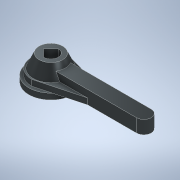
# Autodesk Inventor part: 4-手柄
Saved by Autodesk Inventor 2022 (Build 260153000, 153)
## iProperties
Created: 2023-01-24
Part Number: 4-手柄
Material: 灰口铁
Document SubType Name: Modeling
Designer: Lzy18
Density: 7.15 g/cm^3
Appearance: 灰口铁
Author: Lzy18
Autodesk Inventor part; units mm, degrees
ref_plane "YZ Plane" through (0, 0, 0) normal (1, 0, 0) x (0, 1, 0)
ref_plane "XZ Plane" through (0, 0, 0) normal (0, 1, 0) x (-1, 0, 0)
ref_plane "XY Plane" through (0, 0, 0) normal (0, 0, 1) x (1, 0, 0)
sketch "草图1" plane through (0, 0, 0) normal (0, 1, 0) x (-1, 0, 0)
  arc A0 (0, -13) -> (0, 13) centre (0, 0) ccw
  line L0 (0, 0) -> (-30, 0)
  line L1 (0, -13) -> (-30, -5)
  line L2 (-30, 5) -> (0, 13)
  line L3 (-30, 5) -> (-63, 5)
  line L4 (-63, -5) -> (-30, -5)
  arc A1 (-63, 5) -> (-63, -5) centre (-63, 0) ccw
  dimension "d0" = 26
  dimension "d10" = 10
  constraints: 10 end point, 4 point on circle, 2 centre point, 2 horizontal, 1 coincident, 1 parallel
  measures "d0" diameter of A0
  measures "d10" diameter of A1
extrude "拉伸1" add sketch "草图1" along normal blind 4
sketch "草图2" plane through (0, 0, 0) normal (0, -1, 0) x (1, 0, 0)
  line L0 (30, 5) -> (63, 5) projected
  line L1 (0, 13) -> (30, 5) projected
  arc A0 (0, 13) -> (0, -13) centre (0, 0) ccw projected
  line L2 (30, -5) -> (0, -13) projected
  line L3 (63, -5) -> (30, -5) projected
  circle A1 centre (0, 0) radius 15
  arc A2 (63, -5) -> (63, 5) centre (63, 0) ccw projected
  dimension "d7" = 30
  constraints: 1 centre point, 1 coincident
  measures "d7" diameter of A1
extrude "拉伸2" add sketch "草图2" along normal blind 4 contours A1 L2 A0 L1 | L1 A0 L2 A1
sketch "草图3" plane through (0, 4, 0) normal (0, 1, 0) x (1, 0, 0)
  line L0 (0, -13) -> (30, -5) projected
  line L1 (30, -5) -> (63, -5) projected
  arc A0 (63, -5) -> (63, 5) centre (63, 0) ccw projected
  line L2 (63, 5) -> (30, 5) projected
  line L3 (30, 5) -> (0, 13) projected
  arc A1 (0, 13) -> (0, -13) centre (0, 0) ccw projected
  line L4 (0, -13) -> (30, -5) projected
  line L5 (30, -5) -> (0, -5)
  line L6 (0, -5) -> (0, 5)
  line L7 (0, 5) -> (30, 5)
  constraints: 6 end point, 1 horizontal, 1 parallel, 1 perpendicular
extrude "拉伸3" add sketch "草图3" along normal blind 5 contours L5 L6 L7 L2 A0 L1
sketch "草图4" plane through (0, 0, 0) normal (0, 0, 1) x (1, 0, 0)
  line L0 (0, 0) -> (0, 0) projected
  line L1 (0, 0) -> (0, 4) projected
  line L2 (0, 4) -> (0, 4) projected
  line L3 (0, 0) -> (0, 4) projected
  line L4 (-15, -4) -> (15, -4) projected
  line L5 (11.1585, 0) -> (11.1585, 0) projected
  line L6 (11.1585, 0) -> (11.1585, 0) projected
  line L7 (0, 4) -> (-13, 4) projected
  line L8 (-13, 4) -> (-13, 0)
  line L9 (-15, 0) -> (11.1585, 0) projected
  line L10 (-12, 4) -> (-8, 13)
  line L11 (-8, 13) -> (0, 13)
  line L12 (30, 4) -> (0, 4) projected
  line L13 (0, 13) -> (0, 4)
  dimension "d14" = 1
  dimension "d15" = 9
  dimension "d16" = 8
  constraints: 8 end point, 2 point on line, 1 horizontal, 1 perpendicular, 1 vertical
  measures "d14" distance from line of L8 L10.start
  measures "d15" distance between parallel lines of L7 L11
  measures "d16" distance from line of L13 L10.end
revolve "旋转1" add sketch "草图4" angle 360 about axis through (0, 13, 0) along (0, -1, 0) contours L7 L10 L11 L13
sketch "草图5" plane through (0, 13, 0) normal (0, 1, 0) x (1, 0, 0)
  arc A0 (0, -5) -> (0, 5) centre (0, 0) ccw
  line L0 (0, -5) -> (-5, 0)
  line L1 (-5, 0) -> (0, 5)
  dimension "d18" = 10
  constraints: 4 end point, 2 point on circle, 1 centre point, 1 coincident, 1 perpendicular
  measures "d18" diameter of A0
extrude "拉伸4" cut sketch "草图5" against normal through all
